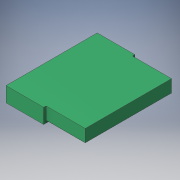
# Autodesk Inventor part: BatteryInBag
Saved by Autodesk Inventor 2016 (Build 200138000, 138)
## iProperties
Created: 2015-09-14
Part Number: BatteryInBag
Material: Generic
Document SubType Name: Modeling
Designer: lachesis
Density: 1 g/cm^3
Appearance: Default
Mass: 513.772 g
Surface Area: 566.003 cm^2
Volume: 513.772 cm^3
Author: lachesis
Autodesk Inventor part; units mm, degrees
ref_plane "YZ Plane" through (0, 0, 0) normal (1, 0, 0) x (0, 1, 0)
ref_plane "XZ Plane" through (0, 0, 0) normal (0, 1, 0) x (-1, 0, 0)
sketch "Sketch1" plane through (0, 0, 0) normal (0, 0, 1) x (1, 0, 0)
  line L0 (0, 11.43) -> (0, -11.43)
  line L1 (0, 13.081) -> (-66.04, 13.081)
  line L2 (-66.04, 13.081) -> (-66.04, -13.081)
  line L3 (-66.04, -13.081) -> (0, -13.081)
  line L4 (0, -13.081) -> (0, 13.081)
  point P0 (0, 0)
  point P1 (0, 0)
  dimension "d1" = 26.162
  dimension "d3" = 66.04
  constraints: 10 end point, 2 midpoint, 2 parallel, 1 coincident, 1 horizontal, 1 perpendicular, 1 point on line
  measures "d1" distance of L1.end L2.end
  measures "d3" distance of L1.start L1.end
extrude "Extrusion1" add sketch "Sketch1" along normal blind 160.02
ref_plane "Work Plane1" through (0, 0, 4.318) normal (0, 0, -1) x (-1, 0, 0)
sketch "Sketch3" plane through (0, 0, 4.318) normal (0, 0, -1) x (-1, 0, 0)
  line L0 (0, 13.081) -> (-68.58, 13.081)
  line L1 (-68.58, 13.081) -> (-68.58, -9.779)
  line L2 (-68.58, -9.779) -> (0, -9.779)
  line L3 (0, -9.779) -> (0, 13.081)
  line L4 (0, -13.081) -> (0, 13.081) projected
  line L5 (66.04, 13.081) -> (66.04, -13.081) projected
  line L6 (0, 13.081) -> (66.04, 13.081) projected
  point P0 (0, 0)
  point P1 (0, 0)
  dimension "d13" = 22.86
  dimension "d14" = 134.62
  constraints: 8 end point, 2 parallel, 1 collinear, 1 horizontal, 1 perpendicular
  measures "d13" distance of L0.end L1.end
  measures "d14" distance between parallel lines of L5 L1
extrude "Extrusion3" add sketch "Sketch3" against normal blind 151.384
fillet "Fillet1" radius 1.27 6 edges at (34.29, -9.779, 4.318) (68.58, -9.779, 80.01) (34.29, -9.779, 155.702) (0, -9.779, 80.01) (0, 1.651, 155.702) (0, 1.651, 4.318)
body "Solid1"
